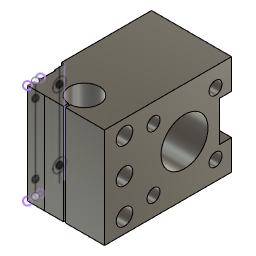
X-End (Autodesk Fusion 360 design; units mm, degrees)
Autodesk Fusion 360 part; units mm, degrees
note: some values were not read from the file. Set by a fixed rule: which sketch regions a step uses.
sketch "Skizze1" plane through (0, 0, 0) normal (0, 0, 1) x (1, 0, 0)
  circle A0 centre (0, 0) radius 7.55
  line L0 (20, -10) -> (-10, -10)
  line L1 (-10, -10) -> (-10, 53.5)
  line L2 (-10, 53.5) -> (20, 53.5)
  line L3 (20, 53.5) -> (20, -10)
  line L4 (0, 0) -> (0, -10)
  line L5 (0, -10) -> (-0.5, -10)
  line L6 (-0.5, -10) -> (0.5, -10)
  line L7 (0.5, -10) -> (0.5, -7.3)
  line L8 (0.5, -7.3) -> (-0.5, -7.3)
  line L9 (-0.5, -7.3) -> (-0.5, -10)
  line L10 (-18, 3.5) -> (-18, -3.5)
  line L11 (-18, 3.5) -> (-18.5, 3.5)
  line L12 (-18, -3.5) -> (-18.5, -3.5)
  line L13 (-18.5, -3.5) -> (-18.5, -10)
  line L14 (-18.5, -10) -> (-10, -10)
  line L15 (-18.5, 3.5) -> (-18.5, 8.5)
  line L16 (-18.5, 8.5) -> (-10, 8.5)
  line L17 (-10, 53.5) -> (-20, 53.5)
  line L18 (-20, 53.5) -> (-20, 8.5)
  line L19 (-20, 8.5) -> (-10, 8.5)
  line L20 (-10, 8.5) -> (-10, 53.5)
  dimension "d1" = 15.1
  dimension "d4" = 20
  dimension "d5" = 10
  dimension "d6" = 10
  dimension "d7" = 63.5
  dimension "d15" = 18
  dimension "d16" = 7
  dimension "d17" = 3.5
  dimension "d18" = 0.5
  dimension "d19" = 0.5
  dimension "d54" = 10
  constraint coincident A0.centre L4.start
  constraint horizontal L0
  constraint vertical L1
  constraint horizontal L2
  constraint vertical L3
  constraint coincident L0 L4.end
  constraint perpendicular L0 L4
  constraint coincident L0 L5.end
  constraint horizontal L6
  constraint vertical L7
  constraint horizontal L8
  constraint vertical L9
  constraint perpendicular L10 L11
  constraint perpendicular L10 L12
  constraint perpendicular L12 L13
  constraint perpendicular L11 L15
  constraint coincident L1 L16.end
  constraint perpendicular L1 L16
  constraint horizontal L17
  constraint vertical L18
  constraint horizontal L19
  constraint vertical L20
  constraint collinear L16 L19
  measures "d1" diameter of A0
  measures "d4" distance of A0.centre L3
  measures "d5" distance of A0.centre L0
  measures "d6" distance of A0.centre L1
  measures "d7" distance of L0.start L2.end
  measures "d15" distance of A0.centre L10
  measures "d16" distance of L10.start L10.end
  measures "d17" vertical distance of A0.centre L10.start
  measures "d18" distance of L10.start L11.end
  measures "d19" distance of L10.end L12.end
  measures "d54" distance of L1.end L17.end
extrude "Extrusion1" add sketch "Skizze1" along normal blind 50 contours A0 L0 L1 L2 L3 L7 L9 L20 | L1 L10 L11 L12 L13 L14 L15 L16 L19 | L1 L16 L17 L18 L19 L20
sketch "Skizze2" plane through (20, 0, 0) normal (1, 0, 0) x (0, 1, 0)
  line L0 (-10, 0) -> (53.5, 0)
  line L1 (53.5, 0) -> (53.5, 50)
  line L2 (53.5, 50) -> (-10, 50)
  line L3 (-10, 50) -> (-10, 0)
  circle A0 centre (0, 25) radius 4.15
  circle A1 centre (30, 25) radius 11.75
  line L4 (14.5, 40.5) -> (45.5, 40.5)
  line L5 (45.5, 40.5) -> (45.5, 9.5)
  line L6 (45.5, 9.5) -> (14.5, 9.5)
  line L7 (14.5, 9.5) -> (14.5, 40.5)
  circle A2 centre (14.5, 40.5) radius 3.25
  circle A3 centre (45.5, 40.5) radius 3.25
  circle A4 centre (45.5, 9.5) radius 3.25
  circle A5 centre (14.5, 9.5) radius 3.25
  circle A6 centre (14.5, 40.5) radius 1.75
  circle A7 centre (45.5, 40.5) radius 1.75
  circle A8 centre (45.5, 9.5) radius 1.75
  circle A9 centre (14.5, 9.5) radius 1.75
  circle A10 centre (0, 7.5) radius 4.15
  circle A11 centre (0, 42.5) radius 4.15
  dimension "d10" = 8.3
  dimension "d11" = 10
  dimension "d42" = 25
  dimension "d55" = 30
  dimension "d56" = 25
  dimension "d57" = 23.5
  dimension "d58" = 31
  dimension "d59" = 31
  dimension "d60" = 15.5
  dimension "d61" = 15.5
  dimension "d62" = 6.5
  dimension "d63" = 3.5
  dimension "d78" = 10
  dimension "d80" = 10
  dimension "d81" = 17.5
  dimension "d82" = 17.5
  constraint horizontal L4
  constraint vertical L5
  constraint horizontal L6
  constraint vertical L7
  constraint coincident L4.start L7.end
  constraint coincident L4.end L5.start
  constraint coincident L5.end L6.start
  constraint coincident L6.end L7.start
  constraint equal A2 A3
  constraint equal A2 A5
  constraint equal A2 A4
  constraint concentric A2 A6
  constraint concentric A3 A7
  constraint concentric A4 A8
  constraint concentric A5 A9
  constraint equal A6 A7
  constraint equal A6 A9
  constraint equal A6 A8
  constraint equal A0 A10
  constraint equal A0 A11
  measures "d10" diameter of A0
  measures "d11" distance of L3 A0.centre
  measures "d42" distance of L0 A0.centre
  measures "d55" horizontal distance of A0.centre A1.centre
  measures "d56" distance of L0 A1.centre
  measures "d57" diameter of A1
  measures "d58" distance of L4.start L4.end
  measures "d59" distance of L4.start L6.end
  measures "d60" distance of A1.centre L4
  measures "d61" distance of A1.centre L7
  measures "d62" diameter of A2
  measures "d63" diameter of A6
  measures "d78" distance of L3 A10.centre
  measures "d80" distance of L3 A11.centre
  measures "d81" distance of A0.centre A11.centre
  measures "d82" distance of A0.centre A10.centre
extrude "Extrusion7" cut sketch "Skizze2" against normal blind 40 contours A1 | L4 L7 A6 | L4 L7 A6 | L4 L5 A7 | L4 L5 A7 | L6 L7 A9 | L6 L7 A9 | L5 L6 A8 | L5 L6 A8
extrude "Extrusion8" cut sketch "Skizze2" against normal blind 35 contours L4 L7 A2 A6 | L4 L7 A2 A6 | L4 L5 A3 A7 | L4 L5 A3 A7 | L6 L7 A5 A9 | L6 L7 A5 A9 | L5 L6 A4 A8 | L5 L6 A4 A8
extrude "Extrusion2" cut sketch "Skizze2" against normal blind 11 contours A0 | A10 | A11
sketch "Skizze3" plane through (0, 0, 50) normal (0, 0, 1) x (-1, 0, 0)
  line L0 (18, -3.5) -> (18, 3.5)
  line L1 (18, 3.5) -> (18.5, 3.5)
  line L2 (18.5, 3.5) -> (18.5, 10)
  line L3 (18.5, 10) -> (10, 10)
  line L4 (10, 10) -> (0.5, 10)
  line L5 (0.5, 10) -> (0.5, 7.5334)
  arc A0 (-0.5, 7.5334) -> (0.5, 7.5334) centre (0, 0) ccw
  line L6 (-0.5, 7.5334) -> (-0.5, 10)
  line L7 (-0.5, 10) -> (-20, 10)
  line L8 (-20, 10) -> (-20, -53.5)
  line L9 (-20, -53.5) -> (20, -53.5)
  line L10 (18.5, -8.5) -> (18.5, -3.5)
  line L11 (18.5, -3.5) -> (18, -3.5)
  line L12 (-20, -53.5) -> (10, -53.5)
  line L13 (10, -53.5) -> (10, -8.5)
  line L14 (-20, -8.5) -> (-20, -53.5)
  arc A1 (-10, -8.5) -> (10, -8.5) centre (0, 0) ccw
  line L15 (-10, -8.5) -> (-20, -8.5)
  line L16 (20, -53.5) -> (20, -8.5)
  line L17 (20, -8.5) -> (18.5, -8.5)
  constraint horizontal L12
  constraint vertical L13
  constraint vertical L14
  constraint coincident L13.end A1.end
  constraint coincident L8.end L9.start
  constraint concentric A0 A1
  constraint perpendicular L8 L15
sketch "Skizze5" plane through (0, 53.5, 0) normal (0, 1, 0) x (-1, 0, 0)
  line L0 (-20, 50) -> (-20, 0)
  line L1 (-20, 0) -> (20, 0)
  line L2 (-20, 25) -> (-13, 25)
  line L3 (-13, 25) -> (-13, 29.75)
  line L4 (-13, 25) -> (-13, 20.25)
  circle A0 centre (-13, 29.75) radius 1.15
  circle A1 centre (-13, 20.25) radius 1.15
  line L5 (20, 50) -> (-20, 50)
  line L6 (20, 0) -> (20, 50)
  dimension "d23" = 7
  dimension "d24" = 4.75
  dimension "d25" = 2.3
  dimension "d26" = 2.3
  constraint midpoint L0 L2.start
  constraint perpendicular L0 L2
  constraint perpendicular L2 L3
  constraint perpendicular L2 L4
  constraint equal L3 L4
  constraint coincident L3.end A0.centre
  constraint coincident L4.end A1.centre
  measures "d23" distance of L2.start L2.end
  measures "d24" distance of L2.end L3.end
  measures "d25" diameter of A0
  measures "d26" diameter of A1
extrude "Extrusion4" cut sketch "Skizze5" against normal blind 11 contours A0 | A1
sketch "Skizze6" plane through (-18.5, 0, 0) normal (-1, 0, 0) x (0, -1, 0)
  line L0 (-8.5, 0) -> (-3.5, 0)
  line L1 (-3.5, 0) -> (-3.5, 50)
  line L2 (-3.5, 50) -> (-8.5, 50)
  line L3 (-6, 50) -> (-6, 0)
  line L4 (6, 50) -> (6, 0)
  circle A0 centre (-6, 42.5) radius 1.5
  circle A1 centre (-6, 7.5) radius 1.5
  circle A2 centre (6, 7.5) radius 1.5
  circle A3 centre (6, 42.5) radius 1.5
  line L5 (3.5, 50) -> (10, 50)
  line L6 (3.5, 0) -> (10, 0)
  line L7 (-8.5, 50) -> (-8.5, 0)
  circle A4 centre (-6, 42.5) radius 3.25
  circle A5 centre (-6, 7.5) radius 3.25
  dimension "d29" = 12
  dimension "d30" = 3
  dimension "d31" = 3
  dimension "d32" = 3
  dimension "d33" = 3
  dimension "d35" = 7.5
  dimension "d36" = 7.5
  dimension "d37" = 7.5
  dimension "d38" = 7.5
  dimension "d73" = 6.5
  dimension "d74" = 6.5
  constraint midpoint L2 L3.start
  constraint midpoint L0 L3.end
  constraint parallel L1 L4
  constraint coincident L3 A0.centre
  constraint coincident L3 A1.centre
  constraint coincident L4 A2.centre
  constraint coincident L4 A3.centre
  constraint concentric A0 A4
  constraint concentric A1 A5
  measures "d29" distance of L3 L4
  measures "d31" diameter of A1
  measures "d32" diameter of A2
  measures "d33" diameter of A3
  measures "d35" distance of A3.centre L5
  measures "d36" distance of L2 A0.centre
  measures "d37" distance of A2.centre L6
  measures "d38" distance of L0 A1.centre
  measures "d74" diameter of A5
extrude "Extrusion5" cut sketch "Skizze6" against normal blind 7 contours L3 A1 | L3 A1 | L3 A0 | L3 A0 | L4 A3 | L4 A3 | L4 A2 | L4 A2
sketch "Skizze9" plane through (0, 53.5, 0) normal (0, 1, 0) x (-1, 0, 0)
  circle A0 centre (-13, 29.75) radius 1.15
  circle A1 centre (-13, 20.25) radius 1.15
  line L0 (-20, 0) -> (20, 0)
  line L1 (20, 0) -> (20, 50)
  line L2 (20, 50) -> (-20, 50)
  line L3 (-20, 50) -> (-20, 0)
  line L4 (-20, 35) -> (-5, 35)
  line L5 (-5, 35) -> (-5, 15)
  line L6 (-5, 15) -> (-20, 15)
  line L7 (-20, 15) -> (-20, 35)
  line L8 (-20, 40.5) -> (-20, 9.5)
  point P0 (-20, 25)
  dimension "d68" = 15
  dimension "d69" = 20
  dimension "d70" = 10
  constraint horizontal L4
  constraint vertical L5
  constraint horizontal L6
  constraint vertical L7
  constraint collinear L7 L8
  measures "d68" distance of L4.start L4.end
  measures "d69" distance of L4.start L6.end
  measures "d70" distance of L4 P0
extrude "Extrusion9" cut sketch "Skizze9" against normal blind 6 contours L3 L4 L5 L6 L7 L8
sketch "Skizze10" plane through (0, 0, 0) normal (0, 0, 1) x (1, 0, 0)
equation "d60 = ( 31 / 2 ) * 1 mm"
equation "d61 = ( 31 / 2 ) * 1 mm"
